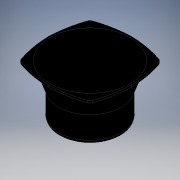
# Autodesk Inventor part: sub
Saved by Autodesk Inventor 2017 (Build 210142000, 142)
## iProperties
Created: 2019-01-31
Part Number: sub
Material: Generic
Document SubType Name: Modeling
Designer: Mitch
Density: 1 g/cm^3
Appearance: Black
Author: Mitch
Autodesk Inventor part; units mm, degrees
ref_plane "YZ Plane" through (0, 0, 0) normal (1, 0, 0) x (0, 1, 0)
ref_plane "XY Plane" through (0, 0, 0) normal (0, 0, 1) x (1, 0, 0)
sketch "Sketch1" plane through (0, 0, 0) normal (0, 1, 0) x (-1, 0, 0)
  circle A0 centre (0, 0) radius 61.9125
  dimension "d0" = 123.825
  constraints: 1 centre point, 1 coincident
  measures "d0" diameter of A0
ref_plane "Work Plane1" through (0, -38.1, 0) normal (0, 1, 0) x (-1, 0, 0)
sketch "Sketch2" plane through (0, -38.1, 0) normal (0, 1, 0) x (-1, 0, 0)
  circle A0 centre (0, 0) radius 48.5775
  dimension "d2" = 97.155
  constraints: 1 centre point, 1 coincident
  measures "d2" diameter of A0
loft "Loft1" add profiles "Sketch1", "Sketch2"
sketch "Sketch3" plane through (0, -38.1, 0) normal (0, -1, 0) x (1, 0, 0)
  circle A0 centre (0, 0) radius 48.5775 projected
extrude "Extrusion1" add sketch "Sketch3" along normal blind 40.64
fillet "Fillet1" radius 6.35 1 edges at (-48.5775, -78.74, 0)
sketch "Sketch4" plane through (0, 0, 0) normal (0, 1, 0) x (1, 0, 0)
  circle A0 centre (0, 0) radius 61.9125 projected
  arc A1 (-54.2856, 54.2856) -> (-64.5795, 0) centre (112.4399, -5.4483) ccw
  line L0 (0, 61.9125) -> (0, -61.9125)
  arc A2 (0, 64.5795) -> (-54.2856, 54.2856) centre (5.4483, -112.4399) ccw
  arc A3 (0, -64.5795) -> (54.2856, -54.2856) centre (-5.4483, 112.4399) ccw
  arc A4 (54.2856, -54.2856) -> (64.5795, 0) centre (-112.4399, 5.4483) ccw
  arc A5 (64.5795, 0) -> (54.2856, 54.2856) centre (-112.4399, -5.4483) ccw
  arc A6 (54.2856, 54.2856) -> (0, 64.5795) centre (-5.4483, -112.4399) ccw
  arc A7 (-64.5795, 0) -> (-54.2856, -54.2856) centre (112.4399, 5.4483) ccw
  arc A8 (-54.2856, -54.2856) -> (0, -64.5795) centre (5.4483, 112.4399) ccw
  circle A9 centre (0, 0) radius 61.9125
  constraints: 16 point on circle, 9 centre point, 5 symmetric about line, 2 end point, 1 coincident, 1 concentric, 4 other
extrude "Extrusion2" add sketch "Sketch4" against normal blind 3.175
fillet "Fillet2" radius 6.35 4 edges at (-54.2856, -1.5875, 54.2856) (54.2856, -1.5875, 54.2856) (54.2856, -1.5875, -54.2856) (-54.2856, -1.5875, -54.2856)
body "Solid1"
